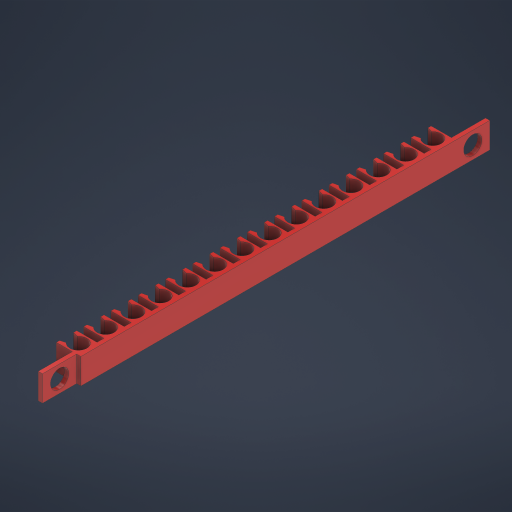
# Autodesk Inventor part: Hose Clamp
Saved by Autodesk Inventor 2024 (Build 280153000, 153)
## iProperties
Created: 2023-05-24
Part Number: Hose Clamp
Material: Generic
Document SubType Name: Modeling
Designer: cfangmeier3
Density: 1 g/cm^3
Appearance: Default
Author: cfangmeier3
Autodesk Inventor part; units mm, degrees
ref_plane "YZ Plane" through (0, 0, 0) normal (1, 0, 0) x (0, 1, 0)
ref_plane "XZ Plane" through (0, 0, 0) normal (0, 1, 0) x (-1, 0, 0)
ref_plane "XY Plane" through (0, 0, 0) normal (0, 0, 1) x (1, 0, 0)
sketch "Sketch1" plane through (0, 0, 0) normal (0, 1, 0) x (-1, 0, 0)
  line L0 (0, 71.12) -> (0, -71.12)
  line L1 (1.5875, 71.12) -> (9.144, 71.12)
  line L2 (9.144, 71.12) -> (9.144, 69.85)
  line L3 (9.144, 64.77) -> (9.144, 63.5)
  line L4 (9.144, 69.85) -> (7.1724, 69.3584)
  line L5 (9.144, 64.77) -> (7.1724, 65.2616)
  arc A0 (7.1724, 69.3584) -> (7.1724, 65.2616) centre (4.7465, 67.31) ccw
  line L6 (9.144, 63.5) -> (1.5875, 63.5)
  line L7 (1.5875, 63.5) -> (1.5875, 60.96)
  line L8 (1.5875, 53.34) -> (1.5875, 50.8)
  line L9 (9.144, 53.34) -> (1.5875, 53.34)
  line L10 (9.144, 54.61) -> (9.144, 53.34)
  line L11 (9.144, 59.69) -> (7.1724, 59.1984)
  arc A1 (7.1724, 59.1984) -> (7.1724, 55.1016) centre (4.7465, 57.15) ccw
  line L12 (1.5875, 60.96) -> (9.144, 60.96)
  line L13 (9.144, 60.96) -> (9.144, 59.69)
  line L14 (9.144, 54.61) -> (7.1724, 55.1016)
  line L15 (1.5875, 43.18) -> (1.5875, 40.64)
  line L16 (9.144, 43.18) -> (1.5875, 43.18)
  line L17 (9.144, 44.45) -> (9.144, 43.18)
  line L18 (9.144, 49.53) -> (7.1724, 49.0384)
  arc A2 (7.1724, 49.0384) -> (7.1724, 44.9416) centre (4.7465, 46.99) ccw
  line L19 (1.5875, 50.8) -> (9.144, 50.8)
  line L20 (9.144, 50.8) -> (9.144, 49.53)
  line L21 (9.144, 44.45) -> (7.1724, 44.9416)
  line L22 (1.5875, 33.02) -> (1.5875, 30.48)
  line L23 (9.144, 33.02) -> (1.5875, 33.02)
  line L24 (9.144, 34.29) -> (9.144, 33.02)
  line L25 (9.144, 39.37) -> (7.1724, 38.8784)
  arc A3 (7.1724, 38.8784) -> (7.1724, 34.7816) centre (4.7465, 36.83) ccw
  line L26 (1.5875, 40.64) -> (9.144, 40.64)
  line L27 (9.144, 40.64) -> (9.144, 39.37)
  line L28 (9.144, 34.29) -> (7.1724, 34.7816)
  line L29 (1.5875, 22.86) -> (1.5875, 20.32)
  line L30 (9.144, 22.86) -> (1.5875, 22.86)
  line L31 (9.144, 24.13) -> (9.144, 22.86)
  line L32 (9.144, 29.21) -> (7.1724, 28.7184)
  arc A4 (7.1724, 28.7184) -> (7.1724, 24.6216) centre (4.7465, 26.67) ccw
  line L33 (1.5875, 30.48) -> (9.144, 30.48)
  line L34 (9.144, 30.48) -> (9.144, 29.21)
  line L35 (9.144, 24.13) -> (7.1724, 24.6216)
  line L36 (1.5875, 12.7) -> (1.5875, 10.16)
  line L37 (9.144, 12.7) -> (1.5875, 12.7)
  line L38 (9.144, 13.97) -> (9.144, 12.7)
  line L39 (9.144, 19.05) -> (7.1724, 18.5584)
  arc A5 (7.1724, 18.5584) -> (7.1724, 14.4616) centre (4.7465, 16.51) ccw
  line L40 (1.5875, 20.32) -> (9.144, 20.32)
  line L41 (9.144, 20.32) -> (9.144, 19.05)
  line L42 (9.144, 13.97) -> (7.1724, 14.4616)
  line L43 (1.5875, 2.54) -> (1.5875, 0)
  line L44 (9.144, 2.54) -> (1.5875, 2.54)
  line L45 (9.144, 3.81) -> (9.144, 2.54)
  line L46 (9.144, 8.89) -> (7.1724, 8.3984)
  arc A6 (7.1724, 8.3984) -> (7.1724, 4.3016) centre (4.7465, 6.35) ccw
  line L47 (1.5875, 10.16) -> (9.144, 10.16)
  line L48 (9.144, 10.16) -> (9.144, 8.89)
  line L49 (9.144, 3.81) -> (7.1724, 4.3016)
  line L50 (1.5875, -7.62) -> (1.5875, -10.16)
  line L51 (9.144, -7.62) -> (1.5875, -7.62)
  line L52 (9.144, -6.35) -> (9.144, -7.62)
  line L53 (9.144, -1.27) -> (7.1724, -1.7616)
  arc A7 (7.1724, -1.7616) -> (7.1724, -5.8584) centre (4.7465, -3.81) ccw
  line L54 (1.5875, 0) -> (9.144, 0)
  line L55 (9.144, 0) -> (9.144, -1.27)
  line L56 (9.144, -6.35) -> (7.1724, -5.8584)
  line L57 (1.5875, -17.78) -> (1.5875, -20.32)
  line L58 (9.144, -17.78) -> (1.5875, -17.78)
  line L59 (9.144, -16.51) -> (9.144, -17.78)
  line L60 (9.144, -11.43) -> (7.1724, -11.9216)
  arc A8 (7.1724, -11.9216) -> (7.1724, -16.0184) centre (4.7465, -13.97) ccw
  line L61 (1.5875, -10.16) -> (9.144, -10.16)
  line L62 (9.144, -10.16) -> (9.144, -11.43)
  line L63 (9.144, -16.51) -> (7.1724, -16.0184)
  line L64 (1.5875, -27.94) -> (1.5875, -30.48)
  line L65 (9.144, -27.94) -> (1.5875, -27.94)
  line L66 (9.144, -26.67) -> (9.144, -27.94)
  line L67 (9.144, -21.59) -> (7.1724, -22.0816)
  arc A9 (7.1724, -22.0816) -> (7.1724, -26.1784) centre (4.7465, -24.13) ccw
  line L68 (1.5875, -20.32) -> (9.144, -20.32)
  line L69 (9.144, -20.32) -> (9.144, -21.59)
  line L70 (9.144, -26.67) -> (7.1724, -26.1784)
  line L71 (1.5875, -38.1) -> (1.5875, -40.64)
  line L72 (9.144, -38.1) -> (1.5875, -38.1)
  line L73 (9.144, -36.83) -> (9.144, -38.1)
  line L74 (9.144, -31.75) -> (7.1724, -32.2416)
  arc A10 (7.1724, -32.2416) -> (7.1724, -36.3384) centre (4.7465, -34.29) ccw
  line L75 (1.5875, -30.48) -> (9.144, -30.48)
  line L76 (9.144, -30.48) -> (9.144, -31.75)
  line L77 (9.144, -36.83) -> (7.1724, -36.3384)
  line L78 (1.5875, -48.26) -> (1.5875, -50.8)
  line L79 (9.144, -48.26) -> (1.5875, -48.26)
  line L80 (9.144, -46.99) -> (9.144, -48.26)
  line L81 (9.144, -41.91) -> (7.1724, -42.4016)
  arc A11 (7.1724, -42.4016) -> (7.1724, -46.4984) centre (4.7465, -44.45) ccw
  line L82 (1.5875, -40.64) -> (9.144, -40.64)
  line L83 (9.144, -40.64) -> (9.144, -41.91)
  line L84 (9.144, -46.99) -> (7.1724, -46.4984)
  line L85 (1.5875, -58.42) -> (1.5875, -60.96)
  line L86 (9.144, -58.42) -> (1.5875, -58.42)
  line L87 (9.144, -57.15) -> (9.144, -58.42)
  line L88 (9.144, -52.07) -> (7.1724, -52.5616)
  arc A12 (7.1724, -52.5616) -> (7.1724, -56.6584) centre (4.7465, -54.61) ccw
  line L89 (1.5875, -50.8) -> (9.144, -50.8)
  line L90 (9.144, -50.8) -> (9.144, -52.07)
  line L91 (9.144, -57.15) -> (7.1724, -56.6584)
  line L92 (1.5875, -68.58) -> (1.5875, -71.12)
  line L93 (9.144, -68.58) -> (1.5875, -68.58)
  line L94 (9.144, -67.31) -> (9.144, -68.58)
  line L95 (9.144, -62.23) -> (7.1724, -62.7216)
  arc A13 (7.1724, -62.7216) -> (7.1724, -66.8184) centre (4.7465, -64.77) ccw
  line L96 (1.5875, -60.96) -> (9.144, -60.96)
  line L97 (9.144, -60.96) -> (9.144, -62.23)
  line L98 (9.144, -67.31) -> (7.1724, -66.8184)
  line L99 (0, 71.12) -> (1.5875, 71.12)
  line L100 (3.175, 71.12) -> (1.5875, 71.12)
  line L101 (1.5875, 71.12) -> (1.5875, 83.82)
  line L102 (1.5875, 83.82) -> (3.175, 83.82)
  line L103 (3.175, 83.82) -> (3.175, 71.12)
  line L104 (1.5875, -71.12) -> (1.5875, -81.28)
  line L105 (1.5875, -81.28) -> (0, -81.28)
  line L106 (0, -81.28) -> (0, -71.12)
  point P0 (0, 0)
  dimension "d1" = 7.5565
  dimension "d5" = 104
  dimension "d6" = 104
  dimension "d7" = 3.175
  dimension "d8" = 2.032
  dimension "d9" = 1.5875
  dimension "d10" = 2.54
  dimension "d11" = 7.62
  dimension "d12" = 1.27
  dimension "d16" = 10.16
  dimension "d25" = 142.24
  dimension "d26" = 71.12
  dimension "d27" = 12.7
  dimension "d28" = 1.5875
  dimension "d29" = 1.5875
  dimension "d41" = 12.7
  constraints: 214 end point, 28 point on circle, 14 centre point, 6 vertical, 4 horizontal, 3 perpendicular, 2 equal length, 2 horizontal alignment, 2 parallel, 1 midpoint, 1 point on line, 1 vertical alignment, 234 other
  measures "d1" distance of L1.start L1.end
  measures "d5" angle of L4 L2
  measures "d6" angle of L5 L3
  measures "d7" radius of A0
  measures "d8" distance of L2.end L4.end
  measures "d9" distance from line of L0 L6.end
  measures "d10" distance of L6.end L7.end
  measures "d11" distance between parallel lines of L1 L6
  measures "d12" distance of L1.end L2.end
  measures "d16" distance of L7.end L8.end
  measures "d25" distance of L0.start L0.end
  measures "d26" distance of L0.end point (0, 0)
  measures "d27" distance of L102.end L100.start
  measures "d28" distance of L101.end L102.end
  measures "d29" distance of L0.start L100.end
  measures "d41" distance between parallel lines of L105 L93
extrude "Extrusion1" add sketch "Sketch1" along normal blind 9.525
sketch "Sketch2" plane through (0, 0, 71.12) normal (1, 0, 0) x (0, 0, -1)
  line L0 (0, 0) -> (152.4, 0) projected
  line L1 (-12.7, 0) -> (-12.7, 9.525) projected
  point P0 (71.12, 0)
  point P1 (146.05, 4.7625)
  point P2 (-6.35, 4.7625)
  point P3 (152.4, 9.525)
  dimension "d31" = 4.7625
  dimension "d42" = 152.4
  dimension "d43" = 165.1
  dimension "d44" = 6.35
  constraints: 1 horizontal alignment
  measures "d31" distance from line of L0 point (146.05, 4.763)
  measures "d42" distance of point (-6.35, 4.763) point (146.05, 4.763)
  measures "d43" distance of L1.end point (152.4, 9.525)
  measures "d44" distance from line of L1 point (-6.35, 4.763)
hole "Hole1" at (0, 4.7625, -74.93) at (0, 4.7625, 77.47) direction (-1, 0, 0) diameter 6.7564 end through all clearance for "Flat Head Machine Screw (82)" size "1/4" standard "Ansi Unified Screw Threads"
equation "\"d6\" = d5"
body "Solid1"
